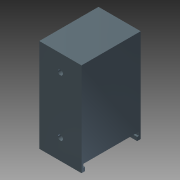
# Autodesk Inventor part: Lead Box
Saved by Autodesk Inventor 2015 SP1 (Build 190203100, 203)
## iProperties
Created: 2015-03-04
Part Number: Lead Box
Material: Lead
Document SubType Name: Modeling
Designer: Andrew
Density: 11.34 g/cm^3
Appearance: Lead
Author: Andrew
Autodesk Inventor part; units mm, degrees
ref_plane "YZ Plane" through (0, 0, 0) normal (1, 0, 0) x (0, 1, 0)
ref_plane "XZ Plane" through (0, 0, 0) normal (0, 1, 0) x (-1, 0, 0)
ref_plane "XY Plane" through (0, 0, 0) normal (0, 0, 1) x (1, 0, 0)
sketch "Sketch1" plane through (0, 0, 0) normal (0, 0, 1) x (1, 0, 0)
  line L0 (-15.5, 23) -> (15.5, 23)
  line L1 (15.5, 23) -> (15.5, -23)
  line L2 (15.5, -23) -> (-15.5, -23)
  line L3 (-15.5, -23) -> (-15.5, 23)
  line L4 (-26.145, 0) -> (26.145, 0) projected
  line L5 (0, 36.645) -> (0, -36.645) projected
  line L6 (18.675, 26.175) -> (-18.675, 26.175)
  line L7 (-18.675, 26.175) -> (-18.675, -26.175)
  line L8 (-18.675, -26.175) -> (18.675, -26.175)
  line L9 (18.675, -26.175) -> (18.675, 26.175)
  point P0 (0, 0)
  dimension "d0" = 46
  dimension "d1" = 31
  dimension "d2" = 3.175
  constraints: 16 end point, 4 parallel, 2 perpendicular, 1 horizontal, 5 other
  measures "d0" distance between parallel lines of L2 L0
  measures "d1" distance between parallel lines of L1 L3
  measures "d2" distance between parallel lines of L0 L6
extrude "Extrusion1" add sketch "Sketch1" along normal mid plane 73 contours L3 L4 L7 L6 L5 L0 | L5 L6 L9 L4 L1 L0 | L3 L2 L5 L8 L7 L4 | L4 L9 L8 L5 L2 L1
sketch "Sketch2" plane through (-18.675, 26.175, 36.5) normal (0, 1, 0) x (1, 0, 0)
  line L0 (0, 73) -> (0, 0) projected
  line L1 (37.35, 0) -> (0, 0) projected
  line L2 (37.35, 0) -> (37.35, 73) projected
  line L3 (0, 73) -> (37.35, 73) projected
  circle A0 centre (18.675, 37.53) radius 10.575
  point P0 (18.675, 36.5)
  dimension "d6" = 1.03
  dimension "d7" = 21.15
  constraints: 1 centre point
  measures "d6" distance of A0.centre point (18.675, 36.5)
  measures "d7" diameter of A0
extrude "Extrusion2" cut sketch "Sketch2" against normal up to surface (3.175 mm away) contours A0
sketch "Sketch3" plane through (0, 0, 36.5) normal (0, 0, 1) x (1, 0, 0)
  line L0 (15.5, 23) -> (15.5, -23) projected
  line L1 (15.5, -23) -> (-15.5, -23) projected
  line L2 (-15.5, -23) -> (-15.5, 23) projected
  line L3 (-15.5, 23) -> (15.5, 23) projected
  line L4 (18.675, 26.175) -> (-18.675, 26.175) projected
  line L5 (-18.675, 26.175) -> (-18.675, -26.175) projected
  line L6 (-18.675, -26.175) -> (18.675, -26.175) projected
  line L7 (18.675, -26.175) -> (18.675, 26.175) projected
  point P0 (0, 0)
extrude "Extrusion3" add sketch "Sketch3" along normal blind 3.175 contours L0 L1 L2 L3 | L7 L6 L5 L4
sketch "Sketch4" plane through (0, 0, -36.5) normal (0, 0, -1) x (-1, 0, 0)
  line L0 (-15.5, -23) -> (-15.5, 23) projected
  line L1 (-15.5, 23) -> (15.5, 23) projected
  line L2 (15.5, 23) -> (15.5, -23) projected
  line L3 (15.5, -23) -> (-15.5, -23) projected
  line L4 (18.675, 26.175) -> (-18.675, 26.175) projected
  line L5 (-18.675, 26.175) -> (-18.675, -26.175) projected
  line L6 (-18.675, -26.175) -> (18.675, -26.175) projected
  line L7 (18.675, -26.175) -> (18.675, 26.175) projected
  line L8 (15.5, -23) -> (18.675, -23)
  line L9 (-15.5, -23) -> (-18.675, -23)
  line L10 (-15.5, 23) -> (-18.675, 23)
  line L11 (15.5, 23) -> (18.675, 23)
  point P0 (0, 0)
  constraints: 8 end point, 7 point on line, 1 perpendicular
extrude "Extrusion4" add sketch "Sketch4" along normal blind 6.35 contours L3 L8 L7 L6 L5 L9 | L10 L5 L4 L7 L11 L1 | L2 L11 L7 L8
sketch "Sketch6" plane through (18.675, -23, -36.5) normal (1, 0, 0) x (0, 0, -1)
  line L0 (-76.175, 49.175) -> (6.35, 49.175) projected
  line L1 (-76.175, -3.175) -> (-76.175, 49.175) projected
  line L2 (6.35, -3.175) -> (-76.175, -3.175) projected
  line L3 (6.35, 0) -> (6.35, -3.175) projected
  line L4 (0, 0) -> (6.35, 0) projected
  line L5 (0, 46) -> (0, 0) projected
  line L6 (0, 46) -> (6.35, 46) projected
  line L7 (6.35, 49.175) -> (6.35, 46) projected
  line L8 (0, 0) -> (0, -1.5875)
  line L9 (0, -1.5875) -> (3.175, -1.5875)
  line L10 (3.175, -1.5875) -> (3.175, 0)
  line L11 (-73, 0) -> (6.35, 0) projected
  line L12 (0, 46) -> (0, 47.5875)
  line L13 (0, 47.5875) -> (3.175, 47.5875)
  line L14 (3.175, 47.5875) -> (3.175, 46)
  line L15 (0, 46) -> (6.35, 46) projected
  line L16 (3.175, 0) -> (3.175, 46)
  point P0 (-36.5, 23)
  dimension "d14" = 1.5875
  dimension "d15" = 3.175
  constraints: 14 end point, 3 perpendicular, 3 point on line, 1 collinear, 1 midpoint, 1 vertical
  measures "d14" distance of L9.end L10.end
  measures "d15" distance of L8.end L9.end
extrude "Extrusion5" cut sketch "Sketch6" against normal blind 35.7625 contours L16 L4 L5 L6 | L6 L12 L13 L14 | L10 L9 L8 L4
sketch "Sketch7" plane through (-15.5, -23, -36.5) normal (0, 1, 0) x (1, 0, 0)
  line L0 (34.175, 6.35) -> (34.175, -76.175) projected
  line L1 (-3.175, -76.175) -> (34.175, -76.175) projected
  line L2 (-3.175, 6.35) -> (-3.175, -76.175) projected
  line L3 (34.175, 6.35) -> (-3.175, 6.35) projected
  line L4 (34.175, 3.175) -> (34.175, 0) projected
  line L5 (34.175, 3.175) -> (-1.5875, 3.175) projected
  line L6 (-1.5875, 3.175) -> (-1.5875, 0) projected
  line L7 (34.175, 0) -> (-1.5875, 0) projected
  circle A0 centre (15.5, -11.5) radius 2.25
  circle A1 centre (15.5, -61.5) radius 2.25
  line L8 (15.5, 22.855) -> (15.5, -92.68) projected
  line L9 (41.645, -36.5) -> (-10.645, -36.5) projected
  point P0 (15.5, -36.5)
  dimension "d18" = 4.5
  dimension "d19" = 50
  constraints: 2 centre point, 1 equal radius, 1 point on line, 1 other
  measures "d18" diameter of A0
  measures "d19" distance of A1.centre A0.centre
extrude "Extrusion6" cut sketch "Sketch7" against normal up to surface (3.175 mm away) contours L8 A0 | A0 L8 | L8 A1 | A1 L8
body "Solid1"
